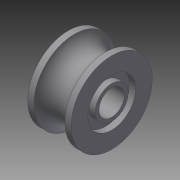
# Autodesk Inventor part: WheelYBottom
Saved by Autodesk Inventor 2015 (Build 190159000, 159)
## iProperties
Created: 2017-01-31
Part Number: WheelYBottom
Material: Generic
Document SubType Name: Modeling
Designer: Ernest
Density: 1 g/cm^3
Appearance: Default
Author: Ernest
Autodesk Inventor part; units mm, degrees
ref_plane "YZ Plane" through (0, 0, 0) normal (1, 0, 0) x (0, 1, 0)
ref_plane "XZ Plane" through (0, 0, 0) normal (0, 1, 0) x (-1, 0, 0)
ref_plane "XY Plane" through (0, 0, 0) normal (0, 0, 1) x (1, 0, 0)
sketch "Sketch1" plane through (0, 0, 0) normal (0, 1, 0) x (-1, 0, 0)
  line L0 (0, 0) -> (0, -4.7) construction
  line L1 (3.5, 0) -> (-3.5, 0) construction
  line L2 (3.5, 0) -> (3.5, -6.55) construction
  line L3 (3.5, -6.55) -> (2.5, -6.55)
  line L4 (-3.5, -6.55) -> (-2.5, -6.55)
  arc A0 (2.5, -6.55) -> (-2.5, -6.55) centre (0, -7.3142) ccw
  line L5 (3.5, -2.05) -> (-3.5, -2.05)
  line L6 (3.5, -2.05) -> (3.5, -6.55)
  line L7 (-3.5, -2.05) -> (-3.5, -6.55)
  dimension "d0" = 4.7
  dimension "d1" = 7
  dimension "d2" = 3.5
  dimension "d3" = 6.55
  dimension "d4" = 1
  dimension "d5" = 1
  dimension "d6" = 2.05
  constraints: 16 end point, 4 horizontal, 3 point on circle, 2 vertical, 1 centre point, 1 parallel, 1 perpendicular, 1 point on line
  measures "d0" distance of L0.start L0.end
  measures "d1" distance of L1.start L1.end
  measures "d2" distance of L0.start L1.end
  measures "d3" distance of L1.start L2.end
  measures "d4" distance of L2.end L3.end
  measures "d5" distance of L4.start L4.end
  measures "d6" distance from line of L0.start L5
revolve "Revolution1" add sketch "Sketch1" angle 360 about axis through (-3.5, 0, 0) along (1, 0, 0)
sketch "Sketch2" plane through (-3.5, 0, 0) normal (-1, 0, 0) x (0, 0, 1)
  circle A0 centre (0, 0) radius 6.55 projected
  circle A1 centre (0, 0) radius 2.05 projected
  circle A2 centre (0, 0) radius 2.65
  circle A3 centre (0, 0) radius 3.85
  point P0 (0, 0)
  dimension "d8" = 5.3
  dimension "d9" = 7.7
  constraints: 2 centre point, 2 coincident
  measures "d8" diameter of A2
  measures "d9" diameter of A3
extrude "Extrusion1" cut sketch "Sketch2" against normal blind 1 contours A3
sketch "Sketch3" plane through (3.5, 0, 0) normal (1, 0, 0) x (0, 0, -1)
  circle A0 centre (0, 0) radius 3.85
  circle A1 centre (0, 0) radius 2.65
  dimension "d12" = 7.7
  dimension "d13" = 5.3
  constraints: 2 centre point, 2 coincident
  measures "d12" diameter of A0
  measures "d13" diameter of A1
extrude "Extrusion2" cut sketch "Sketch3" against normal blind 1
equation "\"d2\" = 0.5 * d1"
body "Solid1"
